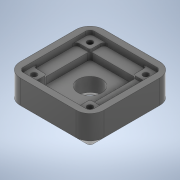
# Autodesk Inventor part: Camera_cover_
Saved by Autodesk Inventor 2020.4 (Build 244396000, 396)
## iProperties
Created: 2021-12-31
Part Number: Camera_cover_
Material: PC/ABS プラスチック
Document SubType Name: Modeling
Designer: Masato Kubotera
Density: 0.357273 g/cm^3
Appearance: 滑らか - 黒
Mass: 20.6565 g
Surface Area: 136.523 cm^2
Volume: 57.8172 cm^3
Description: PLA
Author: Masato Kubotera
Autodesk Inventor part; units mm, degrees
ref_plane "YZ Plane" through (0, 0, 0) normal (1, 0, 0) x (0, 1, 0)
ref_plane "XZ Plane" through (0, 0, 0) normal (0, 1, 0) x (-1, 0, 0)
ref_plane "XY Plane" through (0, 0, 0) normal (0, 0, 1) x (1, 0, 0)
derived "Camera_root_frame_.ipt"
sketch "スケッチ1" plane through (0, 0, 0) normal (0, 0, 1) x (1, 0, 0)
  line L0 (14, 16) -> (-14, 16) construction
  line L1 (-16, 14) -> (-16, -14) construction
  line L2 (-14, -16) -> (14, -16) construction
  line L3 (16, -14) -> (16, 14) construction
  line L4 (16, 16) -> (-16, -16) construction
  line L5 (-16, 16) -> (16, -16) construction
  line L6 (-13, 13) -> (13, 13) construction
  line L7 (13, 13) -> (13, -13) construction
  line L8 (13, -13) -> (-13, -13) construction
  line L9 (-13, -13) -> (-13, 13) construction
  line L10 (-13, 13) -> (13, -13) construction
  line L11 (13, 13) -> (-13, -13) construction
  circle A0 centre (-13, -13) radius 1.1 construction
  line L12 (-16, 0) -> (16, 0) construction
  line L13 (0, 16) -> (0, -16) construction
  circle A1 centre (-13, 13) radius 1.1 construction
  circle A2 centre (13, -13) radius 1.1 construction
  circle A3 centre (13, 13) radius 1.1 construction
  circle A4 centre (-13, -13) radius 2 construction
  circle A5 centre (-13, 13) radius 2 construction
  circle A6 centre (13, -13) radius 2 construction
  circle A7 centre (13, 13) radius 2 construction
  circle A8 centre (0, 0) radius 7.5 construction
  circle A9 centre (-5.5, -9) radius 1.1 construction
  circle A10 centre (-5.5, -9) radius 2 construction
  line L14 (-7.5, -9) -> (-7.5, 7.5) construction
  line L15 (-7.5, 7.5) -> (3.5, 7.5) construction
  line L16 (-3.5, -9) -> (-3.5, -7.5) construction
  circle A11 centre (5.5, 9) radius 2 construction
  line L17 (3.5, 9) -> (3.5, 7.5) construction
  circle A12 centre (5.5, 9) radius 1.1 construction
  line L18 (7.5, 9) -> (7.5, -7.5) construction
  line L19 (7.5, -7.5) -> (-3.5, -7.5) construction
  arc A13 (-16, -14) -> (-14, -16) centre (-14, -14) ccw construction
  arc A14 (14, -16) -> (16, -14) centre (14, -14) ccw construction
  arc A15 (16, 14) -> (14, 16) centre (14, 14) ccw construction
  arc A16 (-14, 16) -> (-16, 14) centre (-14, 14) ccw construction
  line L20 (16, -11.1) -> (15, -11.1) construction
  line L21 (15, -11.1) -> (15, 11.1) construction
  line L22 (16, 11.1) -> (15, 11.1) construction
sketch "スケッチ2" plane through (0, 0, 0) normal (0, 0, 1) x (1, 0, 0)
  line L0 (-22.5, 25) -> (22.5, 25)
  line L1 (25, 22.5) -> (25, -22.5)
  line L2 (22.5, -25) -> (-22.5, -25)
  line L3 (-25, -22.5) -> (-25, 22.5)
  line L4 (-25, 25) -> (25, -25) construction
  line L5 (25, 25) -> (-25, -25) construction
  arc A0 (-22.5, 25) -> (-25, 22.5) centre (-22.5, 22.5) ccw
  arc A1 (-25, -22.5) -> (-22.5, -25) centre (-22.5, -22.5) ccw
  arc A2 (22.5, -25) -> (25, -22.5) centre (22.5, -22.5) ccw
  arc A3 (25, 22.5) -> (22.5, 25) centre (22.5, 22.5) ccw
  line L6 (-25, -22.5) -> (25, -22.5) construction
  line L7 (25, -22.5) -> (25, -17.5)
  line L8 (25, -17.5) -> (-25, -17.5) construction
  line L9 (-25, -17.5) -> (-25, -22.5) construction
  line L10 (-25, -22.5) -> (25, -17.5) construction
  line L11 (25, -22.5) -> (-25, -17.5) construction
  line L12 (-25, -20) -> (25, -20) construction
  line L13 (0, 16) -> (0, -16) construction
  circle A4 centre (-20, -20) radius 1.6
  circle A5 centre (20, -20) radius 1.6
  line L14 (-16, 0) -> (16, 0) construction
  circle A6 centre (-20, 20) radius 1.6
  circle A7 centre (20, 20) radius 1.6
  circle A8 centre (-5.5, -9) radius 2 construction
  circle A9 centre (13, 13) radius 1.1
  circle A10 centre (13, -13) radius 1.1
  circle A11 centre (-13, -13) radius 1.1
  circle A12 centre (-13, 13) radius 1.1
  circle A13 centre (-13, -13) radius 1.55
  circle A14 centre (13, -13) radius 1.55
  circle A15 centre (13, 13) radius 1.55
  circle A16 centre (-13, 13) radius 1.55
  line L15 (-14, -16) -> (14, -16)
  line L16 (-16, 14) -> (-16, -14)
  line L17 (-16, -7.8461) -> (-16, 0)
  line L18 (0, -16) -> (-7.8461, -16)
  arc A17 (-9.8095, -13.619) -> (-13.619, -9.8095) centre (-13, -13) ccw
  arc A18 (-9.8095, -13.619) -> (-7.8461, -16) centre (-7.8461, -14) ccw
  arc A19 (-16, -7.8461) -> (-13.619, -9.8095) centre (-14, -7.8461) ccw
  arc A20 (-13.619, 9.8095) -> (-16, 7.8461) centre (-14, 7.8461) ccw
  arc A21 (-7.8461, 16) -> (-9.8095, 13.619) centre (-7.8461, 14) ccw
  line L19 (-16, 7.8461) -> (-16, 0)
  line L20 (0, 16) -> (-7.8461, 16)
  arc A22 (-13.619, 9.8095) -> (-9.8095, 13.619) centre (-13, 13) ccw
  arc A23 (13.619, -9.8095) -> (16, -7.8461) centre (14, -7.8461) ccw
  arc A24 (7.8461, -16) -> (9.8095, -13.619) centre (7.8461, -14) ccw
  arc A25 (13.619, -9.8095) -> (9.8095, -13.619) centre (13, -13) ccw
  line L21 (16, -7.8461) -> (16, 0)
  line L22 (16, 7.8461) -> (16, 0)
  arc A26 (16, 7.8461) -> (13.619, 9.8095) centre (14, 7.8461) ccw
  arc A27 (9.8095, 13.619) -> (13.619, 9.8095) centre (13, 13) ccw
  arc A28 (9.8095, 13.619) -> (7.8461, 16) centre (7.8461, 14) ccw
  line L23 (0, 16) -> (7.8461, 16)
  line L24 (0, -16) -> (7.8461, -16)
  line L25 (-10, -22.5) -> (10, -22.5) construction
  line L26 (10, -22.5) -> (10, -17.5) construction
  line L27 (10, -17.5) -> (-10, -17.5) construction
  line L28 (-10, -17.5) -> (-10, -22.5) construction
  line L29 (-10, -22.5) -> (10, -17.5) construction
  line L30 (10, -22.5) -> (-10, -17.5) construction
  line L31 (-8.5651, -22.55) -> (8.5651, -22.55)
  line L32 (8.5651, -17.45) -> (-8.5651, -17.45)
  line L33 (-10.05, -22.55) -> (10.05, -17.45) construction
  line L34 (10.05, -22.55) -> (-10.05, -17.45) construction
  arc A29 (-10.05, -21.0651) -> (-8.5651, -22.55) centre (-9.3075, -21.8075) ccw
  arc A30 (-8.5651, -17.45) -> (-10.05, -18.9349) centre (-9.3075, -18.1925) ccw
  arc A31 (10.05, -18.9349) -> (8.5651, -17.45) centre (9.3075, -18.1925) ccw
  arc A32 (8.5651, -22.55) -> (10.05, -21.0651) centre (9.3075, -21.8075) ccw
  line L35 (-10.05, -22.5) -> (-10.05, -22.55)
  line L36 (-10.05, -17.45) -> (-10.05, -17.5)
  line L37 (-10.05, -18.9349) -> (-10.05, -21.0651)
  line L38 (10.05, -22.55) -> (10.05, -22.5)
  line L39 (10.05, -21.0651) -> (10.05, -18.9349)
  line L40 (10.05, -17.5) -> (10.05, -17.45)
  arc A33 (-8.5651, 22.55) -> (-10.05, 21.0651) centre (-9.3075, 21.8075) ccw
  line L41 (-10.05, 18.9349) -> (-10.05, 21.0651)
  arc A34 (-10.05, 18.9349) -> (-8.5651, 17.45) centre (-9.3075, 18.1925) ccw
  line L42 (8.5651, 17.45) -> (-8.5651, 17.45)
  line L43 (-8.5651, 22.55) -> (8.5651, 22.55)
  line L44 (10.05, 21.0651) -> (10.05, 18.9349)
  arc A35 (8.5651, 17.45) -> (10.05, 18.9349) centre (9.3075, 18.1925) ccw
  arc A36 (10.05, 21.0651) -> (8.5651, 22.55) centre (9.3075, 21.8075) ccw
  line L45 (19, -11) -> (22, -11) construction
  line L46 (22, -11) -> (22, 11)
  line L47 (22, 11) -> (19, 11) construction
  line L48 (19, 11) -> (19, -11)
  line L49 (19, -11) -> (22, 11) construction
  line L50 (22, -11) -> (19, 11) construction
  arc A37 (19, -11) -> (22, -11) centre (20.5, -11) ccw
  arc A38 (22, 11) -> (19, 11) centre (20.5, 11) ccw
  arc A39 (-15, -17) -> (-15.5858, -15.5858) centre (-17, -17) ccw
  line L51 (-15, -17) -> (-15, -23)
  arc A40 (-14.9997, -22.9637) -> (-13, -25) centre (-13, -23) ccw
  arc A41 (-15.5858, -15.5858) -> (-17, -15) centre (-17, -17) ccw
  line L52 (-17, -15) -> (-23, -15)
  arc A42 (-25, -13) -> (-22.9637, -14.9997) centre (-23, -13) ccw
  arc A43 (-22.9637, 14.9997) -> (-25, 13) centre (-23, 13) ccw
  line L53 (-17, 15) -> (-23, 15)
  arc A44 (-17, 15) -> (-15.5858, 15.5858) centre (-17, 17) ccw
  arc A45 (-15.5858, 15.5858) -> (-15, 17) centre (-17, 17) ccw
  line L54 (-15, 17) -> (-15, 23)
  arc A46 (-13, 25) -> (-14.9997, 22.9637) centre (-13, 23) ccw
  arc A47 (14.9997, 22.9637) -> (13, 25) centre (13, 23) ccw
  line L55 (15, 17) -> (15, 23)
  arc A48 (15, 17) -> (15.5858, 15.5858) centre (17, 17) ccw
  arc A49 (15.5858, 15.5858) -> (17, 15) centre (17, 17) ccw
  line L56 (17, 15) -> (23, 15)
  arc A50 (25, 13) -> (22.9637, 14.9997) centre (23, 13) ccw
  arc A51 (22.9637, -14.9997) -> (25, -13) centre (23, -13) ccw
  line L57 (17, -15) -> (23, -15)
  arc A52 (17, -15) -> (15.5858, -15.5858) centre (17, -17) ccw
  arc A53 (15.5858, -15.5858) -> (15, -17) centre (17, -17) ccw
  line L58 (15, -17) -> (15, -23)
  arc A54 (13, -25) -> (14.9997, -22.9637) centre (13, -23) ccw
  line L59 (20.5, -12.5) -> (20.5, 12.5) construction
  point P0 (0, 0)
  point P1 (0, -20)
  point P2 (0, -20)
  point P3 (-16, -11.75)
  point P4 (-11.75, -16)
  point P5 (20.5, 0)
  point P6 (20.5, 0)
sketch "スケッチ3" plane through (0, 0, 0) normal (0, 0, 1) x (1, 0, 0)
  arc A0 (-25, -22.5) -> (-22.5, -25) centre (-22.5, -22.5) ccw construction
  line L0 (22.5, -25) -> (-22.5, -25) construction
  circle A1 centre (-20, -20) radius 1.6 construction
  line L1 (-25, -22.5) -> (-25, 22.5) construction
  line L2 (-15, -17) -> (-15, -23) construction
  arc A2 (-14.9997, -22.9637) -> (-13, -25) centre (-13, -23) ccw construction
  arc A3 (-25.5, -22.5) -> (-22.5, -25.5) centre (-22.5, -22.5) ccw
  line L3 (-22.5, -25.5) -> (0, -25.5)
  line L4 (-25.5, -22.5) -> (-25.5, 0)
  line L5 (0, 16) -> (0, -16) construction
  line L6 (-16, 0) -> (16, 0) construction
  arc A4 (-15, -17) -> (-15.5858, -15.5858) centre (-17, -17) ccw construction
  line L7 (25, 25) -> (-25, -25) construction
  arc A5 (-15.5, -17) -> (-15.9393, -15.9393) centre (-17, -17) ccw
  line L8 (-15.5, -17) -> (-15.5, -23)
  arc A6 (-15.5, -23) -> (-13, -25.5) centre (-13, -23) ccw
  circle A7 centre (-20, -20) radius 2
  circle A8 centre (0, 0) radius 8.5
  circle A9 centre (0, 0) radius 7.5 construction
  arc A10 (-15.9393, -15.9393) -> (-17, -15.5) centre (-17, -17) ccw
  line L9 (-17, -15.5) -> (-23, -15.5)
  arc A11 (-25.5, -13) -> (-23, -15.5) centre (-23, -13) ccw
  line L10 (-20, -30) -> (20, -30)
  line L11 (30, -20) -> (30, 20)
  line L12 (20, 30) -> (-20, 30)
  line L13 (-30, 20) -> (-30, -20)
  line L14 (-30, -30) -> (30, 30) construction
  line L15 (30, -30) -> (-30, 30) construction
  arc A12 (-30, -20) -> (-20, -30) centre (-20, -20) ccw
  arc A13 (20, -30) -> (30, -20) centre (20, -20) ccw
  arc A14 (30, 20) -> (20, 30) centre (20, 20) ccw
  arc A15 (-20, 30) -> (-30, 20) centre (-20, 20) ccw
  arc A16 (-22.5, 25.5) -> (-25.5, 22.5) centre (-22.5, 22.5) ccw
  line L16 (-22.5, 25.5) -> (0, 25.5)
  line L17 (-25.5, 22.5) -> (-25.5, 0)
  arc A17 (-15.9393, 15.9393) -> (-15.5, 17) centre (-17, 17) ccw
  line L18 (-15.5, 17) -> (-15.5, 23)
  arc A18 (-13, 25.5) -> (-15.5, 23) centre (-13, 23) ccw
  circle A19 centre (-20, 20) radius 2
  arc A20 (-17, 15.5) -> (-15.9393, 15.9393) centre (-17, 17) ccw
  line L19 (-17, 15.5) -> (-23, 15.5)
  arc A21 (-23, 15.5) -> (-25.5, 13) centre (-23, 13) ccw
  arc A22 (22.5, -25.5) -> (25.5, -22.5) centre (22.5, -22.5) ccw
  line L20 (22.5, -25.5) -> (0, -25.5)
  line L21 (25.5, -22.5) -> (25.5, 0)
  arc A23 (15.9393, -15.9393) -> (15.5, -17) centre (17, -17) ccw
  line L22 (15.5, -17) -> (15.5, -23)
  arc A24 (13, -25.5) -> (15.5, -23) centre (13, -23) ccw
  circle A25 centre (20, -20) radius 2
  arc A26 (17, -15.5) -> (15.9393, -15.9393) centre (17, -17) ccw
  line L23 (17, -15.5) -> (23, -15.5)
  arc A27 (23, -15.5) -> (25.5, -13) centre (23, -13) ccw
  arc A28 (25.5, 22.5) -> (22.5, 25.5) centre (22.5, 22.5) ccw
  line L24 (22.5, 25.5) -> (0, 25.5)
  arc A29 (15.5, 23) -> (13, 25.5) centre (13, 23) ccw
  line L25 (15.5, 17) -> (15.5, 23)
  arc A30 (15.5, 17) -> (15.9393, 15.9393) centre (17, 17) ccw
  line L26 (17, 15.5) -> (23, 15.5)
  arc A31 (15.9393, 15.9393) -> (17, 15.5) centre (17, 17) ccw
  line L27 (25.5, 22.5) -> (25.5, 0)
  arc A32 (25.5, 13) -> (23, 15.5) centre (23, 13) ccw
  circle A33 centre (20, 20) radius 2
  line L28 (-14.5251, -16.5251) -> (14.5251, -16.5251)
  line L29 (16.5251, -14.5251) -> (16.5251, 14.5251)
  line L30 (14.5251, 16.5251) -> (-14.5251, 16.5251)
  line L31 (-16.5251, 14.5251) -> (-16.5251, -14.5251)
  line L32 (-16.5251, -16.5251) -> (16.5251, 16.5251) construction
  line L33 (16.5251, -16.5251) -> (-16.5251, 16.5251) construction
  arc A34 (-16.5251, -14.5251) -> (-14.5251, -16.5251) centre (-14.5251, -14.5251) ccw
  arc A35 (14.5251, -16.5251) -> (16.5251, -14.5251) centre (14.5251, -14.5251) ccw
  arc A36 (16.5251, 14.5251) -> (14.5251, 16.5251) centre (14.5251, 14.5251) ccw
  arc A37 (-14.5251, 16.5251) -> (-16.5251, 14.5251) centre (-14.5251, 14.5251) ccw
  point P0 (25.5, -13)
  point P1 (25.5, 13)
  dimension "d1" = 0.5
  dimension "d2" = 4
  dimension "d3" = 1
  dimension "d4" = 60
  dimension "d5" = 10
  dimension "d14" = 2
  constraints: 56 end point, 56 point on circle, 48 symmetric about line, 33 centre point, 25 point on line, 22 tangent, 6 equal radius, 6 parallel, 5 coincident, 4 midpoint, 3 horizontal, 2 perpendicular, 20 other
  measures "d1" radial gap between concentric circles of A3 A0
  measures "d2" diameter of A7
  measures "d3" radial gap between concentric circles of A8 A9
  measures "d4" distance of L15.end L14.start
  measures "d5" radius of A12
  measures "d14" radius of A34
extrude "押し出し1" add sketch "スケッチ3" against normal blind 25 contours L4 A11 L9 A10 A5 L8 A6 L3 A3 | L4 L17 A21 L19 A20 A37 L31 A34 A10 L9 A11 | A6 L8 A5 A34 L28 A35 A23 L22 A24 L20 L3 | L17 A16 L16 A18 L18 A17 A20 L19 A21 | A24 L22 A23 A26 L23 A27 L21 A22 L20 | A34 L31 A37 L30 A36 L29 A35 L28 | L16 L24 A29 L25 A30 A36 L30 A37 A17 L18 A18 | A27 L23 A26 A35 L29 A36 A31 L26 A32 L27 L21 | L24 A28 L27 A32 L26 A31 A30 L25 A29 | A7 | A12 L13 A15 L12 A14 L11 A13 L10 | A19 | A25 | A33
extrude "押し出し2" cut sketch "スケッチ3" against normal blind 5 contours L4 L17 A21 L19 A20 A37 L31 A34 A10 L9 A11 | A6 L8 A5 A34 L28 A35 A23 L22 A24 L20 L3 | A34 L31 A37 L30 A36 L29 A35 L28 | L16 L24 A29 L25 A30 A36 L30 A37 A17 L18 A18 | A27 L23 A26 A35 L29 A36 A31 L26 A32 L27 L21
extrude "押し出し3" cut sketch "スケッチ3" against normal blind 3 contours L4 A11 L9 A10 A5 L8 A6 L3 A3 | L17 A16 L16 A18 L18 A17 A20 L19 A21 | A24 L22 A23 A26 L23 A27 L21 A22 L20 | L24 A28 L27 A32 L26 A31 A30 L25 A29
extrude "押し出し4" cut sketch "スケッチ3" against normal blind 8 contours A7 | A19 | A25 | A33
extrude "押し出し5" cut sketch "スケッチ3" against normal blind 10 contours A34 L31 A37 L30 A36 L29 A35 L28 | A27 L23 A26 A35 L29 A36 A31 L26 A32 L27 L21
chamfer "面取り1" distance 8 angle 45 8 edges at (30, 0, -25) (27.0711, -27.0711, -25) (0, -30, -25) (-27.0711, -27.0711, -25) (-30, 0, -25) (-27.0711, 27.0711, -25) (0, 30, -25) (27.0711, 27.0711, -25)
chamfer "面取り2" distance 5 angle 45 1 edges at (-8.5, 0, -25)
